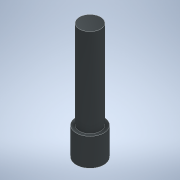
# Autodesk Inventor part: armscrew1
Saved by Autodesk Inventor 2021 (Build 250183000, 183)
## iProperties
Created: 2021-07-07
Part Number: armscrew1
Material: Iron, Gray
Document SubType Name: Modeling
Designer: KAVYA
Density: 7.15 g/cm^3
Appearance: Iron Gray
Author: KAVYA
Autodesk Inventor part; units mm, degrees
ref_plane "YZ Plane" through (0, 0, 0) normal (1, 0, 0) x (0, 1, 0)
ref_plane "XZ Plane" through (0, 0, 0) normal (0, 1, 0) x (-1, 0, 0)
ref_plane "XY Plane" through (0, 0, 0) normal (0, 0, 1) x (1, 0, 0)
sketch "Sketch1" plane through (0, 0, 0) normal (0, 1, 0) x (-1, 0, 0)
  circle A0 centre (0, 0) radius 0.5
  dimension "d0" = 1
  constraints: 1 centre point, 1 coincident
  measures "d0" diameter of A0
extrude "Extrusion1" add sketch "Sketch1" along normal blind 1
sketch "Sketch2" plane through (0, 1, 0) normal (0, 1, 0) x (1, 0, 0)
  circle A0 centre (0, 0) radius 0.381
  dimension "d3" = 0.762
  constraints: 1 centre point, 1 coincident
  measures "d3" diameter of A0
extrude "Extrusion2" add sketch "Sketch2" along normal blind 3.2
sketch "Sketch3" plane through (0, 0, 0) normal (0, -1, 0) x (1, 0, 0)
  line L0 (0.4, 0) -> (0.4, -0.1)
  line L1 (-0.4, -0.1) -> (-0.4, 0)
  line L2 (0.4, 0) -> (0.4, 0.1)
  line L3 (-0.4, 0.1) -> (-0.4, 0)
  line L4 (0, -0.4) -> (0.1, -0.4)
  line L5 (0.1, 0.4) -> (-0.1, 0.4)
  line L6 (-0.1, -0.4) -> (0, -0.4)
  line L7 (-0.1, 0.4) -> (-0.1, 0.1)
  line L8 (-0.1, -0.1) -> (-0.1, -0.4)
  line L9 (0.4, 0.1) -> (0.1, 0.1)
  line L10 (-0.1, 0.1) -> (-0.4, 0.1)
  line L11 (0.1, -0.4) -> (0.1, -0.1)
  line L12 (0.1, 0.1) -> (0.1, 0.4)
  line L13 (0.4, -0.1) -> (0.1, -0.1)
  line L14 (-0.1, -0.1) -> (-0.4, -0.1)
  point P0 (0, 0)
  dimension "d7" = 0.8
  dimension "d8" = 0.1
  dimension "d9" = 0.8
  dimension "d10" = 0.1
  dimension "d11" = 0.1
  dimension "d12" = 0.8
  dimension "d13" = 0.2
  dimension "d14" = 0.8
  constraints: 30 end point, 4 perpendicular, 2 parallel, 1 horizontal, 1 point on line
  measures "d7" distance of L0.end L1.start
  measures "d8" distance of L0.start L0.end
  measures "d9" distance of L3.start L2.end
  measures "d10" distance of L2.end L2.start
  measures "d11" distance of L4.start L4.end
  measures "d12" distance of L4.end L5.start
  measures "d13" distance of L5.start L5.end
  measures "d14" distance of L5.end L6.start
extrude "Extrusion3" cut sketch "Sketch3" against normal blind 0.5
body "Solid1"
